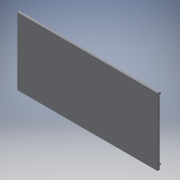
# Autodesk Inventor part: top2b
Saved by Autodesk Inventor 2017 (Build 210142000, 142)
## iProperties
Created: 2016-12-08
Part Number: top2b
Material: Generic
Document SubType Name: Modeling
Designer: SDL
Density: 1 g/cm^3
Appearance: Default
Author: SDL
Autodesk Inventor part; units mm, degrees
ref_plane "YZ Plane" through (0, 0, 0) normal (1, 0, 0) x (0, 1, 0)
ref_plane "XZ Plane" through (0, 0, 0) normal (0, 1, 0) x (-1, 0, 0)
ref_plane "XY Plane" through (0, 0, 0) normal (0, 0, 1) x (1, 0, 0)
sketch "Sketch1" plane through (0, 0, 0) normal (0, 0, 1) x (1, 0, 0)
  line L0 (0, 0) -> (133, 0)
  line L1 (133, 0) -> (133, 64)
  line L2 (133, 64) -> (0, 64)
  line L3 (0, 64) -> (0, 0)
  line L4 (0, 64) -> (0, 62.5)
  line L5 (81.5, 62.5) -> (51.5, 62.5)
  line L6 (51.5, 62.5) -> (51.5, 59.5)
  line L7 (51.5, 59.5) -> (81.5, 59.5)
  line L8 (81.5, 59.5) -> (81.5, 62.5)
  dimension "d0" = 133
  dimension "d1" = 64
  dimension "d6" = 30
  dimension "d7" = 3
  constraints: 18 end point, 4 parallel, 2 horizontal, 2 perpendicular, 1 point on line
  measures "d0" distance of L2.end L1.end
  measures "d1" distance of L1.end L0.end
  measures "d6" distance of L7.end L6.end
  measures "d7" distance of L6.end L5.end
extrude "Extrusion1" add sketch "Sketch1" along normal blind 2 contours L3 L2 L1 L0 | L8 L7 L6 L5
sketch "Sketch2" plane through (0, 0, 2) normal (0, 0, 1) x (1, 0, 0)
  line L0 (133, 64) -> (0, 64) projected
  line L1 (0, 64) -> (0, 0) projected
  line L2 (81.5, 62.5) -> (51.5, 62.5)
  line L3 (51.5, 62.5) -> (51.5, 59)
  line L4 (51.5, 59) -> (81.5, 59)
  line L5 (81.5, 59) -> (81.5, 62.5)
  dimension "d12" = 30
  dimension "d13" = 3.5
  constraints: 8 end point, 2 parallel, 1 horizontal, 1 perpendicular
  measures "d12" distance of L4.end L3.end
  measures "d13" distance of L3.end L2.end
extrude "Extrusion2" add sketch "Sketch2" against normal blind 3
sketch "Sketch3" plane through (0, 0, 0) normal (0, 0, -1) x (-1, 0, 0)
  line L0 (-133, 64) -> (0, 64) projected
  line L1 (0, 64) -> (-6.5, 64)
  line L2 (-133, 0) -> (-133, 64) projected
  circle A0 centre (-6.5, 60.5) radius 1.25
  line L3 (0, 0) -> (-133, 0) projected
  circle A1 centre (-6.5, 3.5) radius 1.25
  circle A2 centre (-130.5, 60.5) radius 1
  line L4 (-133, 0) -> (-130.5, 0)
  line L5 (-133, 0) -> (-130.5, 0) construction
  circle A3 centre (-130.5, 2.5) radius 0.9
  dimension "d19" = 2.5
  dimension "d22" = 2.5
  dimension "d25" = 2
  dimension "d29" = 1.8
  constraints: 6 end point, 4 centre point, 2 collinear, 1 horizontal, 1 point on line
  measures "d19" diameter of A0
  measures "d22" diameter of A1
  measures "d25" diameter of A2
  measures "d29" diameter of A3
extrude "Extrusion3" add sketch "Sketch3" along normal blind 3
sketch "Sketch4" plane through (0, 0, 2) normal (0, 0, 1) x (1, 0, 0)
  line L0 (133, 64) -> (199.5, 64) construction
  line L1 (66.5, 57) -> (62.5, 57)
  line L2 (62.5, 57) -> (62.5, 12)
  line L3 (62.5, 12) -> (127.5, 12)
  line L4 (127.5, 12) -> (127.5, 57)
  line L5 (127.5, 57) -> (62.5, 57)
  point P0 (0, 0)
  dimension "d37" = 65
  dimension "d38" = 45
  constraints: 12 end point, 2 horizontal, 2 perpendicular, 1 collinear, 1 point on line
  measures "d37" distance of L2.end L3.end
  measures "d38" distance of L3.end L4.end
extrude "Extrusion4" cut sketch "Sketch4" against normal blind 2
sketch "Sketch5" plane through (0, 0, 2) normal (0, 0, 1) x (1, 0, 0)
  line L0 (3.5226, 54.2576) -> (52.9878, 54.2576) construction
  line L1 (52.9878, 54.2576) -> (52.9878, 20.7529) construction
  line L2 (52.9878, 20.7529) -> (3.5226, 20.7529) construction
  line L3 (3.5226, 20.7529) -> (3.5226, 54.2576) construction
  line L4 (3.948, 49.9691) -> (3.948, 54.1691)
  line L5 (3.948, 54.1691) -> (6.5756, 54.1691)
  line L6 (6.5756, 54.1691) -> (6.5756, 53.6722)
  line L7 (6.5756, 53.6722) -> (4.5062, 53.6722)
  line L8 (4.5062, 53.6722) -> (4.5062, 52.5218)
  line L9 (4.5062, 52.5218) -> (6.436, 52.5218)
  line L10 (6.436, 52.5218) -> (6.436, 52.0249)
  line L11 (6.436, 52.0249) -> (4.5062, 52.0249)
  line L12 (4.5062, 52.0249) -> (4.5062, 50.4661)
  line L13 (4.5062, 50.4661) -> (6.5756, 50.4661)
  line L14 (6.5756, 50.4661) -> (6.5756, 49.9691)
  line L15 (6.5756, 49.9691) -> (3.948, 49.9691)
  spline S0 degree 2 poles (8.3591, 49.8943) (7.903, 49.8943) (7.2631, 50.0849) (6.9806, 50.221) knots 0 0 0 1 2 2 2
  line L16 (6.9806, 50.221) -> (6.9806, 50.9221)
  line L17 (6.9806, 50.9221) -> (7.0215, 50.9221)
  spline S1 degree 2 poles (7.0215, 50.9221) (7.2971, 50.6635) (7.9949, 50.3776) (8.3182, 50.3776) knots 0 0 0 1 2 2 2
  spline S2 degree 2 poles (8.3182, 50.3776) (8.7811, 50.3776) (9.2542, 50.7622) (9.2542, 51.0787) knots 0 0 0 1 2 2 2
  spline S3 degree 2 poles (9.2542, 51.0787) (9.2542, 51.3306) (9.0057, 51.6437) (8.7369, 51.722) knots 0 0 0 1 2 2 2
  spline S4 degree 2 poles (8.7369, 51.722) (8.5429, 51.7764) (8.2195, 51.8513) (7.9779, 51.9126) knots 0 0 0 1 2 2 2
  spline S5 degree 2 poles (7.9779, 51.9126) (7.76, 51.9704) (7.4163, 52.144) (7.2835, 52.2836) knots 0 0 0 1 2 2 2
  spline S6 degree 2 poles (7.2835, 52.2836) (7.1542, 52.4231) (7.0112, 52.7975) (7.0112, 53.0426) knots 0 0 0 1 2 2 2
  spline S7 degree 2 poles (7.0112, 53.0426) (7.0112, 53.5531) (7.8077, 54.244) (8.4237, 54.244) knots 0 0 0 1 2 2 2
  spline S8 degree 2 poles (8.4237, 54.244) (8.7777, 54.244) (9.404, 54.1045) (9.6728, 53.9717) knots 0 0 0 1 2 2 2
  line L18 (9.6728, 53.9717) -> (9.6728, 53.3046)
  line L19 (9.6728, 53.3046) -> (9.632, 53.3046)
  spline S9 degree 2 poles (9.632, 53.3046) (9.4312, 53.4884) (8.8049, 53.7607) (8.4612, 53.7607) knots 0 0 0 1 2 2 2
  spline S10 degree 2 poles (8.4612, 53.7607) (8.0732, 53.7607) (7.5933, 53.3965) (7.5933, 53.1004) knots 0 0 0 1 2 2 2
  spline S11 degree 2 poles (7.5933, 53.1004) (7.5933, 52.8349) (7.8758, 52.5184) (8.1412, 52.4469) knots 0 0 0 1 2 2 2
  spline S12 degree 2 poles (8.1412, 52.4469) (8.3182, 52.3993) (8.8322, 52.2768) (9.0023, 52.2257) knots 0 0 0 1 2 2 2
  spline S13 degree 2 poles (9.0023, 52.2257) (9.4346, 52.093) (9.8362, 51.5586) (9.8362, 51.1672) knots 0 0 0 1 2 2 2
  spline S14 degree 2 poles (9.8362, 51.1672) (9.8362, 50.9187) (9.6354, 50.4422) (9.455, 50.2755) knots 0 0 0 1 2 2 2
  spline S15 degree 2 poles (9.455, 50.2755) (9.2542, 50.0917) (8.7437, 49.8943) (8.3591, 49.8943) knots 0 0 0 1 2 2 2
  line L20 (10.4046, 49.9691) -> (10.4046, 54.1691)
  line L21 (10.4046, 54.1691) -> (13.0322, 54.1691)
  line L22 (13.0322, 54.1691) -> (13.0322, 53.6722)
  line L23 (13.0322, 53.6722) -> (10.9628, 53.6722)
  line L24 (10.9628, 53.6722) -> (10.9628, 52.5218)
  line L25 (10.9628, 52.5218) -> (12.8926, 52.5218)
  line L26 (12.8926, 52.5218) -> (12.8926, 52.0249)
  line L27 (12.8926, 52.0249) -> (10.9628, 52.0249)
  line L28 (10.9628, 52.0249) -> (10.9628, 50.4661)
  line L29 (10.9628, 50.4661) -> (13.0322, 50.4661)
  line L30 (13.0322, 50.4661) -> (13.0322, 49.9691)
  line L31 (13.0322, 49.9691) -> (10.4046, 49.9691)
  spline S16 degree 2 poles (16.463, 53.7709) (16.3098, 53.7709) (16.0069, 53.696) (15.8605, 53.6382) knots 0 0 0 1 2 2 2
  spline S17 degree 2 poles (15.8605, 53.6382) (15.7244, 53.5803) (15.5236, 53.4578) (15.4453, 53.4033) knots 0 0 0 1 2 2 2
  line L32 (15.4453, 53.4033) -> (15.4112, 53.4033)
  line L33 (15.4112, 53.4033) -> (15.4112, 53.999)
  spline S18 degree 2 poles (15.4112, 53.999) (15.595, 54.0977) (16.2247, 54.2576) (16.5072, 54.2576) knots 0 0 0 1 2 2 2
  spline S19 degree 2 poles (16.5072, 54.2576) (16.7931, 54.2576) (17.2185, 54.1419) (17.3921, 54.0194) knots 0 0 0 1 2 2 2
  spline S20 degree 2 poles (17.3921, 54.0194) (17.5759, 53.8866) (17.7665, 53.502) (17.7665, 53.2434) knots 0 0 0 1 2 2 2
  spline S21 degree 2 poles (17.7665, 53.2434) (17.7665, 52.8962) (17.3104, 52.3721) (16.9905, 52.304) knots 0 0 0 1 2 2 2
  line L34 (16.9905, 52.304) -> (16.9905, 52.2631)
  spline S22 degree 2 poles (16.9905, 52.2631) (17.1232, 52.2359) (17.4262, 52.1134) (17.5555, 51.9909) knots 0 0 0 1 2 2 2
  spline S23 degree 2 poles (17.5555, 51.9909) (17.6848, 51.8717) (17.8482, 51.4905) (17.8482, 51.2148) knots 0 0 0 1 2 2 2
  spline S24 degree 2 poles (17.8482, 51.2148) (17.8482, 50.9324) (17.6542, 50.4525) (17.4772, 50.2687) knots 0 0 0 1 2 2 2
  spline S25 degree 2 poles (17.4772, 50.2687) (17.2934, 50.0781) (16.7727, 49.8807) (16.4425, 49.8807) knots 0 0 0 1 2 2 2
  spline S26 degree 2 poles (16.4425, 49.8807) (16.126, 49.8807) (15.5065, 50.0338) (15.2955, 50.1393) knots 0 0 0 1 2 2 2
  line L35 (15.2955, 50.1393) -> (15.2955, 50.7349)
  line L36 (15.2955, 50.7349) -> (15.3364, 50.7349)
  spline S27 degree 2 poles (15.3364, 50.7349) (15.5134, 50.6056) (16.1124, 50.3674) (16.4085, 50.3674) knots 0 0 0 1 2 2 2
  spline S28 degree 2 poles (16.4085, 50.3674) (16.5821, 50.3674) (16.9292, 50.4763) (17.045, 50.6022) knots 0 0 0 1 2 2 2
  spline S29 degree 2 poles (17.045, 50.6022) (17.1573, 50.7281) (17.2764, 51.0277) (17.2764, 51.2557) knots 0 0 0 1 2 2 2
  spline S30 degree 2 poles (17.2764, 51.2557) (17.2764, 51.4837) (17.1437, 51.7798) (17.0245, 51.8649) knots 0 0 0 1 2 2 2
  spline S31 degree 2 poles (17.0245, 51.8649) (16.9054, 51.95) (16.5821, 52.0147) (16.3915, 52.0147) knots 0 0 0 1 2 2 2
  line L37 (16.3915, 52.0147) -> (16.1532, 52.0147)
  line L38 (16.1532, 52.0147) -> (16.1532, 52.481)
  line L39 (16.1532, 52.481) -> (16.3404, 52.481)
  spline S32 degree 2 poles (16.3404, 52.481) (16.7182, 52.481) (17.1947, 52.8418) (17.1947, 53.1855) knots 0 0 0 1 2 2 2
  spline S33 degree 2 poles (17.1947, 53.1855) (17.1947, 53.3455) (17.0722, 53.5735) (16.9735, 53.6416) knots 0 0 0 1 2 2 2
  spline S34 degree 2 poles (16.9735, 53.6416) (16.868, 53.7131) (16.6093, 53.7709) (16.463, 53.7709) knots 0 0 0 1 2 2 2
  line L40 (21.0714, 49.9691) -> (18.4813, 49.9691)
  line L41 (18.4813, 49.9691) -> (18.4813, 50.5648)
  spline S35 degree 2 poles (18.4813, 50.5648) (18.7604, 50.8268) (19.2573, 51.3136) (19.4955, 51.5756) knots 0 0 0 1 2 2 2
  spline S36 degree 2 poles (19.4955, 51.5756) (19.9754, 52.1032) (20.326, 52.7362) (20.326, 53.0732) knots 0 0 0 1 2 2 2
  spline S37 degree 2 poles (20.326, 53.0732) (20.326, 53.2502) (20.2171, 53.5157) (20.1184, 53.6007) knots 0 0 0 1 2 2 2
  spline S38 degree 2 poles (20.1184, 53.6007) (20.0197, 53.6858) (19.761, 53.7709) (19.6044, 53.7709) knots 0 0 0 1 2 2 2
  spline S39 degree 2 poles (19.6044, 53.7709) (19.4547, 53.7709) (19.1484, 53.696) (19.0088, 53.6382) knots 0 0 0 1 2 2 2
  spline S40 degree 2 poles (19.0088, 53.6382) (18.8897, 53.5905) (18.6685, 53.4544) (18.6004, 53.4067) knots 0 0 0 1 2 2 2
  line L42 (18.6004, 53.4067) -> (18.5698, 53.4067)
  line L43 (18.5698, 53.4067) -> (18.5698, 54.0058)
  spline S41 degree 2 poles (18.5698, 54.0058) (18.7433, 54.0909) (19.3662, 54.2576) (19.6453, 54.2576) knots 0 0 0 1 2 2 2
  spline S42 degree 2 poles (19.6453, 54.2576) (20.2341, 54.2576) (20.8978, 53.6348) (20.8978, 53.1038) knots 0 0 0 1 2 2 2
  spline S43 degree 2 poles (20.8978, 53.1038) (20.8978, 52.8554) (20.7821, 52.4401) (20.68, 52.2631) knots 0 0 0 1 2 2 2
  spline S44 degree 2 poles (20.68, 52.2631) (20.5779, 52.0794) (20.2818, 51.7186) (20.1184, 51.545) knots 0 0 0 1 2 2 2
  spline S45 degree 2 poles (20.1184, 51.545) (19.8529, 51.2557) (19.2028, 50.6362) (19.0088, 50.4559) knots 0 0 0 1 2 2 2
  line L44 (19.0088, 50.4559) -> (21.0714, 50.4559)
  line L45 (21.0714, 50.4559) -> (21.0714, 49.9691)
  spline S46 degree 2 poles (22.7664, 53.7709) (22.6132, 53.7709) (22.3103, 53.696) (22.1639, 53.6382) knots 0 0 0 1 2 2 2
  spline S47 degree 2 poles (22.1639, 53.6382) (22.0278, 53.5803) (21.827, 53.4578) (21.7487, 53.4033) knots 0 0 0 1 2 2 2
  line L46 (21.7487, 53.4033) -> (21.7147, 53.4033)
  line L47 (21.7147, 53.4033) -> (21.7147, 53.999)
  spline S48 degree 2 poles (21.7147, 53.999) (21.8984, 54.0977) (22.5281, 54.2576) (22.8106, 54.2576) knots 0 0 0 1 2 2 2
  spline S49 degree 2 poles (22.8106, 54.2576) (23.0965, 54.2576) (23.5219, 54.1419) (23.6955, 54.0194) knots 0 0 0 1 2 2 2
  spline S50 degree 2 poles (23.6955, 54.0194) (23.8793, 53.8866) (24.0699, 53.502) (24.0699, 53.2434) knots 0 0 0 1 2 2 2
  spline S51 degree 2 poles (24.0699, 53.2434) (24.0699, 52.8962) (23.6138, 52.3721) (23.2939, 52.304) knots 0 0 0 1 2 2 2
  line L48 (23.2939, 52.304) -> (23.2939, 52.2631)
  spline S52 degree 2 poles (23.2939, 52.2631) (23.4266, 52.2359) (23.7296, 52.1134) (23.8589, 51.9909) knots 0 0 0 1 2 2 2
  spline S53 degree 2 poles (23.8589, 51.9909) (23.9882, 51.8717) (24.1516, 51.4905) (24.1516, 51.2148) knots 0 0 0 1 2 2 2
  spline S54 degree 2 poles (24.1516, 51.2148) (24.1516, 50.9324) (23.9576, 50.4525) (23.7806, 50.2687) knots 0 0 0 1 2 2 2
  spline S55 degree 2 poles (23.7806, 50.2687) (23.5968, 50.0781) (23.0761, 49.8807) (22.7459, 49.8807) knots 0 0 0 1 2 2 2
  spline S56 degree 2 poles (22.7459, 49.8807) (22.4294, 49.8807) (21.81, 50.0338) (21.5989, 50.1393) knots 0 0 0 1 2 2 2
  line L49 (21.5989, 50.1393) -> (21.5989, 50.7349)
  line L50 (21.5989, 50.7349) -> (21.6398, 50.7349)
  spline S57 degree 2 poles (21.6398, 50.7349) (21.8168, 50.6056) (22.4158, 50.3674) (22.7119, 50.3674) knots 0 0 0 1 2 2 2
  spline S58 degree 2 poles (22.7119, 50.3674) (22.8855, 50.3674) (23.2326, 50.4763) (23.3484, 50.6022) knots 0 0 0 1 2 2 2
  spline S59 degree 2 poles (23.3484, 50.6022) (23.4607, 50.7281) (23.5798, 51.0277) (23.5798, 51.2557) knots 0 0 0 1 2 2 2
  spline S60 degree 2 poles (23.5798, 51.2557) (23.5798, 51.4837) (23.4471, 51.7798) (23.3279, 51.8649) knots 0 0 0 1 2 2 2
  spline S61 degree 2 poles (23.3279, 51.8649) (23.2088, 51.95) (22.8855, 52.0147) (22.6949, 52.0147) knots 0 0 0 1 2 2 2
  line L51 (22.6949, 52.0147) -> (22.4566, 52.0147)
  line L52 (22.4566, 52.0147) -> (22.4566, 52.481)
  line L53 (22.4566, 52.481) -> (22.6438, 52.481)
  spline S62 degree 2 poles (22.6438, 52.481) (23.0216, 52.481) (23.4981, 52.8418) (23.4981, 53.1855) knots 0 0 0 1 2 2 2
  spline S63 degree 2 poles (23.4981, 53.1855) (23.4981, 53.3455) (23.3756, 53.5735) (23.2769, 53.6416) knots 0 0 0 1 2 2 2
  spline S64 degree 2 poles (23.2769, 53.6416) (23.1714, 53.7131) (22.9127, 53.7709) (22.7664, 53.7709) knots 0 0 0 1 2 2 2
  spline S65 degree 2 poles (6.6028, 45.9878) (6.6028, 45.7155) (6.4088, 45.2254) (6.2352, 45.0553) knots 0 0 0 1 2 2 2
  spline S66 degree 2 poles (6.2352, 45.0553) (6.0174, 44.8408) (5.4286, 44.6196) (4.9793, 44.6196) knots 0 0 0 1 2 2 2
  line L54 (4.9793, 44.6196) -> (4.5062, 44.6196)
  line L55 (4.5062, 44.6196) -> (4.5062, 43.054)
  line L56 (4.5062, 43.054) -> (3.948, 43.054)
  line L57 (3.948, 43.054) -> (3.948, 47.254)
  line L58 (3.948, 47.254) -> (5.0031, 47.254)
  spline S67 degree 2 poles (5.0031, 47.254) (5.3775, 47.254) (5.9017, 47.1314) (6.1025, 46.9919) knots 0 0 0 1 2 2 2
  spline S68 degree 2 poles (6.1025, 46.9919) (6.3373, 46.8319) (6.6028, 46.3384) (6.6028, 45.9878) knots 0 0 0 1 2 2 2
  spline S69 degree 2 poles (6.0208, 45.9708) (6.0208, 46.1886) (5.8711, 46.5086) (5.7179, 46.6107) knots 0 0 0 1 2 2 2
  spline S70 degree 2 poles (5.7179, 46.6107) (5.5852, 46.6992) (5.2312, 46.7706) (4.9691, 46.7706) knots 0 0 0 1 2 2 2
  line L59 (4.9691, 46.7706) -> (4.5062, 46.7706)
  line L60 (4.5062, 46.7706) -> (4.5062, 45.0961)
  line L61 (4.5062, 45.0961) -> (4.8874, 45.0961)
  spline S71 degree 2 poles (4.8874, 45.0961) (5.2278, 45.0961) (5.6464, 45.205) (5.7826, 45.348) knots 0 0 0 1 2 2 2
  spline S72 degree 2 poles (5.7826, 45.348) (5.9085, 45.4739) (6.0208, 45.77) (6.0208, 45.9708) knots 0 0 0 1 2 2 2
  line L62 (8.7641, 45.6373) -> (8.7369, 45.6373)
  spline S73 degree 2 poles (8.7369, 45.6373) (8.6756, 45.6543) (8.5429, 45.6611) (8.451, 45.6611) knots 0 0 0 1 2 2 2
  spline S74 degree 2 poles (8.451, 45.6611) (8.2365, 45.6611) (7.8145, 45.4739) (7.6239, 45.2901) knots 0 0 0 1 2 2 2
  line L63 (7.6239, 45.2901) -> (7.6239, 43.054)
  line L64 (7.6239, 43.054) -> (7.0929, 43.054)
  line L65 (7.0929, 43.054) -> (7.0929, 46.2057)
  line L66 (7.0929, 46.2057) -> (7.6239, 46.2057)
  line L67 (7.6239, 46.2057) -> (7.6239, 45.736)
  spline S75 degree 2 poles (7.6239, 45.736) (7.9132, 45.9946) (8.3454, 46.2057) (8.5497, 46.2057) knots 0 0 0 1 2 2 2
  spline S76 degree 2 poles (8.5497, 46.2057) (8.6313, 46.2057) (8.713, 46.1988) (8.7641, 46.1886) knots 0 0 0 1 2 2 2
  line L68 (8.7641, 46.1886) -> (8.7641, 45.6373)
  spline S77 degree 2 poles (11.766, 44.6298) (11.766, 43.8334) (11.0002, 42.9655) (10.3604, 42.9655) knots 0 0 0 1 2 2 2
  spline S78 degree 2 poles (10.3604, 42.9655) (9.7035, 42.9655) (8.9513, 43.8606) (8.9513, 44.6298) knots 0 0 0 1 2 2 2
  spline S79 degree 2 poles (8.9513, 44.6298) (8.9513, 45.4194) (9.7273, 46.2941) (10.3604, 46.2941) knots 0 0 0 1 2 2 2
  spline S80 degree 2 poles (10.3604, 46.2941) (11.0002, 46.2941) (11.766, 45.4228) (11.766, 44.6298) knots 0 0 0 1 2 2 2
  spline S81 degree 2 poles (11.2181, 44.6298) (11.2181, 45.2424) (10.7722, 45.8381) (10.3604, 45.8381) knots 0 0 0 1 2 2 2
  spline S82 degree 2 poles (10.3604, 45.8381) (9.9485, 45.8381) (9.4993, 45.2424) (9.4993, 44.6298) knots 0 0 0 1 2 2 2
  spline S83 degree 2 poles (9.4993, 44.6298) (9.4993, 44.0342) (9.9485, 43.4215) (10.3604, 43.4215) knots 0 0 0 1 2 2 2
  spline S84 degree 2 poles (10.3604, 43.4215) (10.7688, 43.4215) (11.2181, 44.024) (11.2181, 44.6298) knots 0 0 0 1 2 2 2
  line L69 (13.9681, 46.9306) -> (13.9409, 46.9306)
  spline S85 degree 2 poles (13.9409, 46.9306) (13.8694, 46.9578) (13.604, 47.0055) (13.4984, 47.0055) knots 0 0 0 1 2 2 2
  spline S86 degree 2 poles (13.4984, 47.0055) (13.1649, 47.0055) (12.879, 46.706) (12.879, 46.3112) knots 0 0 0 1 2 2 2
  line L70 (12.879, 46.3112) -> (12.879, 46.2057)
  line L71 (12.879, 46.2057) -> (13.7571, 46.2057)
  line L72 (13.7571, 46.2057) -> (13.7571, 45.7666)
  line L73 (13.7571, 45.7666) -> (12.896, 45.7666)
  line L74 (12.896, 45.7666) -> (12.896, 43.054)
  line L75 (12.896, 43.054) -> (12.3651, 43.054)
  line L76 (12.3651, 43.054) -> (12.3651, 45.7666)
  line L77 (12.3651, 45.7666) -> (12.0077, 45.7666)
  line L78 (12.0077, 45.7666) -> (12.0077, 46.2057)
  line L79 (12.0077, 46.2057) -> (12.3651, 46.2057)
  line L80 (12.3651, 46.2057) -> (12.3651, 46.3112)
  spline S87 degree 2 poles (12.3651, 46.3112) (12.3651, 46.8762) (12.913, 47.4684) (13.4236, 47.4684) knots 0 0 0 1 2 2 2
  spline S88 degree 2 poles (13.4236, 47.4684) (13.5699, 47.4684) (13.8524, 47.4377) (13.9681, 47.4173) knots 0 0 0 1 2 2 2
  line L81 (13.9681, 47.4173) -> (13.9681, 46.9306)
  line L82 (14.9722, 43.054) -> (14.2983, 43.054)
  line L83 (14.2983, 43.054) -> (14.2983, 43.8572)
  line L84 (14.2983, 43.8572) -> (14.9722, 43.8572)
  line L85 (14.9722, 43.8572) -> (14.9722, 43.054)
  line L86 (22.4498, 47.254) -> (21.3947, 43.054)
  line L87 (21.3947, 43.054) -> (20.7685, 43.054)
  line L88 (20.7685, 43.054) -> (19.9142, 46.5392)
  line L89 (19.9142, 46.5392) -> (19.0837, 43.054)
  line L90 (19.0837, 43.054) -> (18.4642, 43.054)
  line L91 (18.4642, 43.054) -> (17.3921, 47.254)
  line L92 (17.3921, 47.254) -> (17.9673, 47.254)
  line L93 (17.9673, 47.254) -> (18.8114, 43.7721)
  line L94 (18.8114, 43.7721) -> (19.6487, 47.254)
  line L95 (19.6487, 47.254) -> (20.2171, 47.254)
  line L96 (20.2171, 47.254) -> (21.0612, 43.7313)
  line L97 (21.0612, 43.7313) -> (21.9018, 47.254)
  line L98 (21.9018, 47.254) -> (22.4498, 47.254)
  spline S89 degree 2 poles (24.2775, 42.9825) (23.5219, 42.9825) (22.6915, 43.83) (22.6915, 44.6128) knots 0 0 0 1 2 2 2
  spline S90 degree 2 poles (22.6915, 44.6128) (22.6915, 45.382) (23.4981, 46.2941) (24.1482, 46.2941) knots 0 0 0 1 2 2 2
  spline S91 degree 2 poles (24.1482, 46.2941) (24.4409, 46.2941) (24.8936, 46.124) (25.0604, 45.9436) knots 0 0 0 1 2 2 2
  spline S92 degree 2 poles (25.0604, 45.9436) (25.2305, 45.7632) (25.4109, 45.2424) (25.4109, 44.8647) knots 0 0 0 1 2 2 2
  line L99 (25.4109, 44.8647) -> (25.4109, 44.5753)
  line L100 (25.4109, 44.5753) -> (23.2292, 44.5753)
  spline S93 degree 2 poles (23.2292, 44.5753) (23.2292, 44.0274) (23.7806, 43.4454) (24.2707, 43.4454) knots 0 0 0 1 2 2 2
  spline S94 degree 2 poles (24.2707, 43.4454) (24.4443, 43.4454) (24.7813, 43.5236) (24.9174, 43.5849) knots 0 0 0 1 2 2 2
  spline S95 degree 2 poles (24.9174, 43.5849) (25.0604, 43.653) (25.2578, 43.7721) (25.3224, 43.8266) knots 0 0 0 1 2 2 2
  line L101 (25.3224, 43.8266) -> (25.3531, 43.8266)
  line L102 (25.3531, 43.8266) -> (25.3531, 43.248)
  spline S96 degree 2 poles (25.3531, 43.248) (25.2612, 43.2105) (24.9821, 43.1016) (24.8732, 43.071) knots 0 0 0 1 2 2 2
  spline S97 degree 2 poles (24.8732, 43.071) (24.72, 43.0267) (24.4681, 42.9825) (24.2775, 42.9825) knots 0 0 0 1 2 2 2
  spline S98 degree 2 poles (24.8936, 44.9804) (24.8868, 45.1948) (24.7983, 45.5079) (24.7132, 45.6134) knots 0 0 0 1 2 2 2
  spline S99 degree 2 poles (24.7132, 45.6134) (24.6213, 45.7326) (24.332, 45.8585) (24.1176, 45.8585) knots 0 0 0 1 2 2 2
  spline S100 degree 2 poles (24.1176, 45.8585) (23.9065, 45.8585) (23.6104, 45.7326) (23.4879, 45.61) knots 0 0 0 1 2 2 2
  spline S101 degree 2 poles (23.4879, 45.61) (23.3688, 45.4841) (23.2463, 45.1812) (23.2292, 44.9804) knots 0 0 0 1 2 2 2
  line L103 (23.2292, 44.9804) -> (24.8936, 44.9804)
  spline S102 degree 2 poles (26.7996, 42.9791) (26.483, 42.9791) (25.9351, 43.1493) (25.7547, 43.2446) knots 0 0 0 1 2 2 2
  line L104 (25.7547, 43.2446) -> (25.7547, 43.8402)
  line L105 (25.7547, 43.8402) -> (25.7819, 43.8402)
  spline S103 degree 2 poles (25.7819, 43.8402) (25.85, 43.7857) (26.0338, 43.6564) (26.1869, 43.5849) knots 0 0 0 1 2 2 2
  spline S104 degree 2 poles (26.1869, 43.5849) (26.3197, 43.5202) (26.6464, 43.4249) (26.82, 43.4249) knots 0 0 0 1 2 2 2
  spline S105 degree 2 poles (26.82, 43.4249) (26.9459, 43.4249) (27.2352, 43.4828) (27.3033, 43.5305) knots 0 0 0 1 2 2 2
  spline S106 degree 2 poles (27.3033, 43.5305) (27.402, 43.5951) (27.4905, 43.7415) (27.4905, 43.8912) knots 0 0 0 1 2 2 2
  spline S107 degree 2 poles (27.4905, 43.8912) (27.4905, 44.0784) (27.2863, 44.2724) (27.0242, 44.3371) knots 0 0 0 1 2 2 2
  spline S108 degree 2 poles (27.0242, 44.3371) (26.9221, 44.3609) (26.5954, 44.429) (26.4558, 44.4664) knots 0 0 0 1 2 2 2
  spline S109 degree 2 poles (26.4558, 44.4664) (26.095, 44.5719) (25.7683, 45.0076) (25.7683, 45.3173) knots 0 0 0 1 2 2 2
  spline S110 degree 2 poles (25.7683, 45.3173) (25.7683, 45.7462) (26.4116, 46.2805) (26.9425, 46.2805) knots 0 0 0 1 2 2 2
  spline S111 degree 2 poles (26.9425, 46.2805) (27.2046, 46.2805) (27.7356, 46.1512) (27.9159, 46.0525) knots 0 0 0 1 2 2 2
  line L106 (27.9159, 46.0525) -> (27.9159, 45.4841)
  line L107 (27.9159, 45.4841) -> (27.8887, 45.4841)
  spline S112 degree 2 poles (27.8887, 45.4841) (27.6845, 45.6475) (27.1876, 45.8347) (26.9323, 45.8347) knots 0 0 0 1 2 2 2
  spline S113 degree 2 poles (26.9323, 45.8347) (26.6702, 45.8347) (26.3095, 45.6134) (26.3095, 45.3922) knots 0 0 0 1 2 2 2
  spline S114 degree 2 poles (26.3095, 45.3922) (26.3095, 45.1914) (26.5239, 44.9974) (26.7621, 44.9361) knots 0 0 0 1 2 2 2
  spline S115 degree 2 poles (26.7621, 44.9361) (26.8779, 44.9055) (27.1706, 44.8442) (27.3305, 44.8068) knots 0 0 0 1 2 2 2
  spline S116 degree 2 poles (27.3305, 44.8068) (27.6777, 44.7183) (28.0317, 44.3133) (28.0317, 43.9627) knots 0 0 0 1 2 2 2
  spline S117 degree 2 poles (28.0317, 43.9627) (28.0317, 43.7585) (27.8717, 43.3977) (27.7151, 43.265) knots 0 0 0 1 2 2 2
  spline S118 degree 2 poles (27.7151, 43.265) (27.5484, 43.1254) (27.1229, 42.9791) (26.7996, 42.9791) knots 0 0 0 1 2 2 2
  spline S119 degree 2 poles (29.4782, 42.9927) (29.0459, 42.9927) (28.5592, 43.4862) (28.5592, 44.0206) knots 0 0 0 1 2 2 2
  line L108 (28.5592, 44.0206) -> (28.5592, 45.7666)
  line L109 (28.5592, 45.7666) -> (28.2018, 45.7666)
  line L110 (28.2018, 45.7666) -> (28.2018, 46.2057)
  line L111 (28.2018, 46.2057) -> (28.5592, 46.2057)
  line L112 (28.5592, 46.2057) -> (28.5592, 47.111)
  line L113 (28.5592, 47.111) -> (29.0902, 47.111)
  line L114 (29.0902, 47.111) -> (29.0902, 46.2057)
  line L115 (29.0902, 46.2057) -> (30.067, 46.2057)
  line L116 (30.067, 46.2057) -> (30.067, 45.7666)
  line L117 (30.067, 45.7666) -> (29.0902, 45.7666)
  line L118 (29.0902, 45.7666) -> (29.0902, 44.2656)
  spline S120 degree 2 poles (29.0902, 44.2656) (29.0902, 44.0274) (29.1072, 43.7653) (29.1651, 43.653) knots 0 0 0 1 2 2 2
  spline S121 degree 2 poles (29.1651, 43.653) (29.2127, 43.5543) (29.4271, 43.4556) (29.6109, 43.4556) knots 0 0 0 1 2 2 2
  spline S122 degree 2 poles (29.6109, 43.4556) (29.7403, 43.4556) (29.9819, 43.5339) (30.0364, 43.5577) knots 0 0 0 1 2 2 2
  line L119 (30.0364, 43.5577) -> (30.067, 43.5577)
  line L120 (30.067, 43.5577) -> (30.067, 43.0812)
  spline S123 degree 2 poles (30.067, 43.0812) (29.9172, 43.0403) (29.6109, 42.9927) (29.4782, 42.9927) knots 0 0 0 1 2 2 2
  spline S124 degree 2 poles (31.8266, 42.9825) (31.0711, 42.9825) (30.2406, 43.83) (30.2406, 44.6128) knots 0 0 0 1 2 2 2
  spline S125 degree 2 poles (30.2406, 44.6128) (30.2406, 45.382) (31.0472, 46.2941) (31.6973, 46.2941) knots 0 0 0 1 2 2 2
  spline S126 degree 2 poles (31.6973, 46.2941) (31.99, 46.2941) (32.4427, 46.124) (32.6095, 45.9436) knots 0 0 0 1 2 2 2
  spline S127 degree 2 poles (32.6095, 45.9436) (32.7796, 45.7632) (32.96, 45.2424) (32.96, 44.8647) knots 0 0 0 1 2 2 2
  line L121 (32.96, 44.8647) -> (32.96, 44.5753)
  line L122 (32.96, 44.5753) -> (30.7783, 44.5753)
  spline S128 degree 2 poles (30.7783, 44.5753) (30.7783, 44.0274) (31.3297, 43.4454) (31.8198, 43.4454) knots 0 0 0 1 2 2 2
  spline S129 degree 2 poles (31.8198, 43.4454) (31.9934, 43.4454) (32.3304, 43.5236) (32.4665, 43.5849) knots 0 0 0 1 2 2 2
  spline S130 degree 2 poles (32.4665, 43.5849) (32.6095, 43.653) (32.8069, 43.7721) (32.8715, 43.8266) knots 0 0 0 1 2 2 2
  line L123 (32.8715, 43.8266) -> (32.9022, 43.8266)
  line L124 (32.9022, 43.8266) -> (32.9022, 43.248)
  spline S131 degree 2 poles (32.9022, 43.248) (32.8103, 43.2105) (32.5312, 43.1016) (32.4223, 43.071) knots 0 0 0 1 2 2 2
  spline S132 degree 2 poles (32.4223, 43.071) (32.2691, 43.0267) (32.0172, 42.9825) (31.8266, 42.9825) knots 0 0 0 1 2 2 2
  spline S133 degree 2 poles (32.4427, 44.9804) (32.4359, 45.1948) (32.3474, 45.5079) (32.2623, 45.6134) knots 0 0 0 1 2 2 2
  spline S134 degree 2 poles (32.2623, 45.6134) (32.1704, 45.7326) (31.8811, 45.8585) (31.6667, 45.8585) knots 0 0 0 1 2 2 2
  spline S135 degree 2 poles (31.6667, 45.8585) (31.4557, 45.8585) (31.1595, 45.7326) (31.037, 45.61) knots 0 0 0 1 2 2 2
  spline S136 degree 2 poles (31.037, 45.61) (30.9179, 45.4841) (30.7954, 45.1812) (30.7783, 44.9804) knots 0 0 0 1 2 2 2
  line L125 (30.7783, 44.9804) -> (32.4427, 44.9804)
  line L126 (35.1689, 45.6373) -> (35.1417, 45.6373)
  spline S137 degree 2 poles (35.1417, 45.6373) (35.0805, 45.6543) (34.9477, 45.6611) (34.8558, 45.6611) knots 0 0 0 1 2 2 2
  spline S138 degree 2 poles (34.8558, 45.6611) (34.6414, 45.6611) (34.2194, 45.4739) (34.0288, 45.2901) knots 0 0 0 1 2 2 2
  line L127 (34.0288, 45.2901) -> (34.0288, 43.054)
  line L128 (34.0288, 43.054) -> (33.4978, 43.054)
  line L129 (33.4978, 43.054) -> (33.4978, 46.2057)
  line L130 (33.4978, 46.2057) -> (34.0288, 46.2057)
  line L131 (34.0288, 46.2057) -> (34.0288, 45.736)
  spline S139 degree 2 poles (34.0288, 45.736) (34.3181, 45.9946) (34.7503, 46.2057) (34.9545, 46.2057) knots 0 0 0 1 2 2 2
  spline S140 degree 2 poles (34.9545, 46.2057) (35.0362, 46.2057) (35.1179, 46.1988) (35.1689, 46.1886) knots 0 0 0 1 2 2 2
  line L132 (35.1689, 46.1886) -> (35.1689, 45.6373)
  line L133 (37.2383, 46.9306) -> (37.2111, 46.9306)
  spline S141 degree 2 poles (37.2111, 46.9306) (37.1396, 46.9578) (36.8741, 47.0055) (36.7686, 47.0055) knots 0 0 0 1 2 2 2
  spline S142 degree 2 poles (36.7686, 47.0055) (36.4351, 47.0055) (36.1492, 46.706) (36.1492, 46.3112) knots 0 0 0 1 2 2 2
  line L134 (36.1492, 46.3112) -> (36.1492, 46.2057)
  line L135 (36.1492, 46.2057) -> (37.0273, 46.2057)
  line L136 (37.0273, 46.2057) -> (37.0273, 45.7666)
  line L137 (37.0273, 45.7666) -> (36.1662, 45.7666)
  line L138 (36.1662, 45.7666) -> (36.1662, 43.054)
  line L139 (36.1662, 43.054) -> (35.6352, 43.054)
  line L140 (35.6352, 43.054) -> (35.6352, 45.7666)
  line L141 (35.6352, 45.7666) -> (35.2779, 45.7666)
  line L142 (35.2779, 45.7666) -> (35.2779, 46.2057)
  line L143 (35.2779, 46.2057) -> (35.6352, 46.2057)
  line L144 (35.6352, 46.2057) -> (35.6352, 46.3112)
  spline S143 degree 2 poles (35.6352, 46.3112) (35.6352, 46.8762) (36.1832, 47.4684) (36.6937, 47.4684) knots 0 0 0 1 2 2 2
  spline S144 degree 2 poles (36.6937, 47.4684) (36.8401, 47.4684) (37.1226, 47.4377) (37.2383, 47.4173) knots 0 0 0 1 2 2 2
  line L145 (37.2383, 47.4173) -> (37.2383, 46.9306)
  spline S145 degree 2 poles (38.7869, 42.9825) (38.0313, 42.9825) (37.2009, 43.83) (37.2009, 44.6128) knots 0 0 0 1 2 2 2
  spline S146 degree 2 poles (37.2009, 44.6128) (37.2009, 45.382) (38.0075, 46.2941) (38.6576, 46.2941) knots 0 0 0 1 2 2 2
  spline S147 degree 2 poles (38.6576, 46.2941) (38.9503, 46.2941) (39.403, 46.124) (39.5698, 45.9436) knots 0 0 0 1 2 2 2
  spline S148 degree 2 poles (39.5698, 45.9436) (39.7399, 45.7632) (39.9203, 45.2424) (39.9203, 44.8647) knots 0 0 0 1 2 2 2
  line L146 (39.9203, 44.8647) -> (39.9203, 44.5753)
  line L147 (39.9203, 44.5753) -> (37.7386, 44.5753)
  spline S149 degree 2 poles (37.7386, 44.5753) (37.7386, 44.0274) (38.29, 43.4454) (38.7801, 43.4454) knots 0 0 0 1 2 2 2
  spline S150 degree 2 poles (38.7801, 43.4454) (38.9537, 43.4454) (39.2907, 43.5236) (39.4268, 43.5849) knots 0 0 0 1 2 2 2
  spline S151 degree 2 poles (39.4268, 43.5849) (39.5698, 43.653) (39.7672, 43.7721) (39.8318, 43.8266) knots 0 0 0 1 2 2 2
  line L148 (39.8318, 43.8266) -> (39.8625, 43.8266)
  line L149 (39.8625, 43.8266) -> (39.8625, 43.248)
  spline S152 degree 2 poles (39.8625, 43.248) (39.7706, 43.2105) (39.4915, 43.1016) (39.3826, 43.071) knots 0 0 0 1 2 2 2
  spline S153 degree 2 poles (39.3826, 43.071) (39.2294, 43.0267) (38.9775, 42.9825) (38.7869, 42.9825) knots 0 0 0 1 2 2 2
  spline S154 degree 2 poles (39.403, 44.9804) (39.3962, 45.1948) (39.3077, 45.5079) (39.2226, 45.6134) knots 0 0 0 1 2 2 2
  spline S155 degree 2 poles (39.2226, 45.6134) (39.1307, 45.7326) (38.8414, 45.8585) (38.627, 45.8585) knots 0 0 0 1 2 2 2
  spline S156 degree 2 poles (38.627, 45.8585) (38.4159, 45.8585) (38.1198, 45.7326) (37.9973, 45.61) knots 0 0 0 1 2 2 2
  spline S157 degree 2 poles (37.9973, 45.61) (37.8782, 45.4841) (37.7557, 45.1812) (37.7386, 44.9804) knots 0 0 0 1 2 2 2
  line L150 (37.7386, 44.9804) -> (39.403, 44.9804)
  line L151 (40.9993, 43.054) -> (40.4683, 43.054)
  line L152 (40.4683, 43.054) -> (40.4683, 47.4412)
  line L153 (40.4683, 47.4412) -> (40.9993, 47.4412)
  line L154 (40.9993, 47.4412) -> (40.9993, 43.054)
  line L155 (44.202, 43.054) -> (43.6711, 43.054)
  line L156 (43.6711, 43.054) -> (43.6711, 43.3739)
  spline S158 degree 2 poles (43.6711, 43.3739) (43.5485, 43.2718) (43.3681, 43.1356) (43.2456, 43.0778) knots 0 0 0 1 2 2 2
  spline S159 degree 2 poles (43.2456, 43.0778) (43.1333, 43.0233) (42.8916, 42.9655) (42.7317, 42.9655) knots 0 0 0 1 2 2 2
  spline S160 degree 2 poles (42.7317, 42.9655) (42.473, 42.9655) (42.0373, 43.1799) (41.8842, 43.3875) knots 0 0 0 1 2 2 2
  spline S161 degree 2 poles (41.8842, 43.3875) (41.731, 43.5951) (41.5608, 44.2078) (41.5608, 44.606) knots 0 0 0 1 2 2 2
  spline S162 degree 2 poles (41.5608, 44.606) (41.5608, 45.0212) (41.7753, 45.6271) (41.9625, 45.8551) knots 0 0 0 1 2 2 2
  spline S163 degree 2 poles (41.9625, 45.8551) (42.136, 46.0593) (42.6228, 46.2941) (42.8916, 46.2941) knots 0 0 0 1 2 2 2
  spline S164 degree 2 poles (42.8916, 46.2941) (43.1265, 46.2941) (43.4771, 46.1886) (43.6711, 46.0797) knots 0 0 0 1 2 2 2
  line L157 (43.6711, 46.0797) -> (43.6711, 47.4412)
  line L158 (43.6711, 47.4412) -> (44.202, 47.4412)
  line L159 (44.202, 47.4412) -> (44.202, 43.054)
  line L160 (43.6711, 43.8198) -> (43.6711, 45.6407)
  spline S165 degree 2 poles (43.6711, 45.6407) (43.4736, 45.736) (43.1605, 45.8074) (42.9801, 45.8074) knots 0 0 0 1 2 2 2
  spline S166 degree 2 poles (42.9801, 45.8074) (42.5717, 45.8074) (42.1088, 45.1948) (42.1088, 44.6162) knots 0 0 0 1 2 2 2
  spline S167 degree 2 poles (42.1088, 44.6162) (42.1088, 44.058) (42.4628, 43.4692) (42.8542, 43.4692) knots 0 0 0 1 2 2 2
  spline S168 degree 2 poles (42.8542, 43.4692) (43.0618, 43.4692) (43.4839, 43.6598) (43.6711, 43.8198) knots 0 0 0 1 2 2 2
  point P0 (0, 0)
  constraints: 2 other
extrude "Extrusion5" add sketch "Sketch5" along normal blind 2
fillet "Fillet1" radius 2 8 edges at (95, 57, 2) (62.5, 34.5, 2) (95, 12, 2) (127.5, 34.5, 2) (66.5, 64, 2) (133, 32, 2) (66.5, 0, 2) (0, 32, 2)
body "Solid1"
